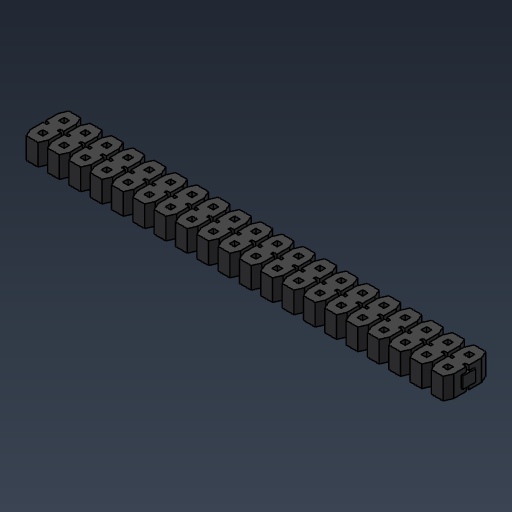
# Autodesk Inventor part: TSM-120-01-T-DV-P_body
Saved by Autodesk Inventor 2023.1 (Build 271208000, 208)
## iProperties
Category: PARTsolutions
Company: SAMTEC
Created: 2015-08-01
Part Number: TSM-120-01-T-DV-P_body
Catalog Web Link: www.cadenas.de
Description: TSM Series Body-TSM Series - (2,54 mm) .100" Surface Mount Terminal .025" Square Post Header
Vendor: SAMTEC
Document SubType Name: Modeling
Designer: PARTuser1
Manufacturer: SAMTEC
Mass: 0.492067 g
Surface Area: 13.1563 cm^2
Volume: 0.492067 cm^3
Density: 1 g/cm^3
Material: Allgemein
Appearance: PSOLRGB-127-127-127
PSOL_IDENT_0: {$CADENAS_DATA\23d-libs\samtec\modelling\tsm\parts\tsm_body.prj},251 {VTYP=3D},{NB=TSM-120-01-T-DV-P
PSOL_IDENT_1: _body},{LINA=TSM-120-01-T-DV-P_body},{NN=TSM Series Body},{DATE=20.05.2015 13:50:20},{GEOMDATE=20.05
PSOL_IDENT_2: .2015 06:27:00},{VERSION=},{LINEID=10},{LINESUBID=-1},{WBVAR=POS,LS,ROW,PLOPT,LCOPT,AOPT,SLOPT,POLOP
PSOL_IDENT_3: T,POPT,TROPT,KOPT}  {NB=TSM-120-01-T-DV-P_body},{LINA=TSM-120-01-T-DV-P_body},{KT=DUMMY},{PN=TSM-120
PSOL_IDENT_4: -01-T-DV-P},{SERIES=TSM},{POS=20},{POSPN=20},{LS=-01},{LSALG= '-01','-01','-02','-02','-03','-03','-
PSOL_IDENT_5: 04','-04' ,'-05','-05 (Non-standard option -  Please contact SAMTEC)' },{ROW=-DV},{ROWALG= '-SV','-S
PSOL_IDENT_6: V - Single Vertical', '-SH','-SH - Single Horizontal', '-DV' ,'-DV - Double Vertical' ,'-DV-S' ,'-DV
PSOL_IDENT_7: -S - Double Vertical Molded End Shrouds (Non-standard option -  Please contact SAMTEC)', '-DH', '-DH
PSOL_IDENT_8: - Double Horizontal' ,  '-MT','-MT - Mixed Technology','-EM','-EM - Edge Mount', '-TM','-TM - Tripl
PSOL_IDENT_9: e Mixed Technology'  },{PLOPT=-T},{PLOPTALG= '-T','-T - Matte Tin on Entire Pin','-S','-S - 30micro\
PSOL_IDENT_10: " Selective Gold in Contact Area, Matte Tin on Tail','-G','-G - 10micro\" Selective Gold in Contact
PSOL_IDENT_11: Area, 3micro\" Selective Gold on Tail','-L','-L - 10micro\" Selective Gold in Contact Area, Matte Ti
PSOL_IDENT_12: n on Tail','-TL','-TL - Tin/Lead (90/10) on Entire Pin','-STL','-STL - 30micro\" Selective Gold in C
PSOL_IDENT_13: ontact Area, Tin/Lead (90/10) on Tail','-F','-F - 3micro\" Selective Gold in Contact Area, Matte Tin
PSOL_IDENT_14: on Tail','-H','-H - 30micro\" Selective Gold in Contact Area, Matte Tin on Tail','-TM','-TM - Matte
PSOL_IDENT_15: Tin on Entire Pin','-SM','-SM - 30micro\" Selective Gold in Contact Area, Matte Tin on Tail','-LM','
PSOL_IDENT_16: -LM - 10micro\" Selective Gold in Contact Area, Matte Tin on Tail','-FM','-FM - 3micro\" Selective G
PSOL_IDENT_17: old in Contact Area, Matte Tin on Tail','-SS','-SS - 30micro\" Stripe Selective Gold in Contact Area
PSOL_IDENT_18: , Matte Tin on Tail' },{LCOPT=},{LCOPTALG= '','Not Selected','-LC','-LC - Locking Clip' },{AOPT=},{A
PSOL_IDENT_19: OPTALG= '','Not Selected','-A' , '-A - Alignment Pin'  },{SLOPT=},{SLOPTALG= '','Not Available' },{P
PSOL_IDENT_20: OLOPT=},{POLOPTALG= '','Not Selected','001','001','002','002','003','003','004','004','005','005','0
PSOL_IDENT_21: 06','006','007','007','008','008','009','009','010','010','011','011','012','012','013','013','014','
PSOL_IDENT_22: 014','015','015','016','016','017','017','018','018','019','019','020','020','021','021','022','022'
PSOL_IDENT_23: ,'023','023','024','024','025','025','026','026','027','027','028','028','029','029','030','030','03
PSOL_IDENT_24: 1','031','032','032','033','033','034','034','035','035','036','036','037','037','038','038','039','
PSOL_IDENT_25: 039','040','040' },{POLOPTMAX=480},{POLOPTMAX2='001','001','002','002','003','003','004','004','005'
PSOL_IDENT_26: ,'005','006','006','007','007','008','008','009','009','010','010','011','011','012','012','013','01
PSOL_IDENT_27: 3','014','014','015','015','016','016','017','017','018','018','019','019','020','020','021','021','
PSOL_IDENT_28: 022','022','023','023','024','024','025','025','026','026','027','027','028','028','029','029','030'
PSOL_IDENT_29: ,'030','031','031','032','032','033','033','034','034','035','035','036','036','037','037','038','03
PSOL_IDENT_30: 8','039','039','040','040'},{POLARIZE='001','001','002','002','003','003','004','004','005','005','0
PSOL_IDENT_31: 06','006','007','007','008','008','009','009','010','010','011','011','012','012','013','013','014','
PSOL_IDENT_32: 014','015','015','016','016','017','017','018','018','019','019','020','020','021','021','022','022'
PSOL_IDENT_33: ,'023','023','024','024','025','025','026','026','027','027','028','028','029','029','030','030','03
PSOL_IDENT_34: 1','031','032','032','033','033','034','034','035','035','036','036','037','037','038','038','039','
PSOL_IDENT_35: 039','040','040','041','041','042','042','043','043','044','044','045','045','046','046','047','047'
PSOL_IDENT_36: ,'048','048','049','049','050','050','051','051','052','052','053','053','054','054','055','055','05
PSOL_IDENT_37: 6','056','057','057','058','058','059','059','060','060','061','061','062','062','063','063','064','
PSOL_IDENT_38: 064','065','065','066','066','067','067','068','068','069','069','070','070','071','071','072','072'
PSOL_IDENT_39: ,'073','073','074','074','075','075','076','076','077','077','078','078','079','079','080','080','08
PSOL_IDENT_40: 1','081','082','082','083','083','084','084','085','085','086','086','087','087','088','088','089','
PSOL_IDENT_41: 089','090','090','091','091','092','092','093','093','094','094','095','095','096','096','097','097'
PSOL_IDENT_42: ,'098','098','099','099','100','100','101','101','102','102','103','103','104','104','105','105','10
PSOL_IDENT_43: 6','106','107','107','108','108','109','109','110','110','111','111','112','112','113','113','114','
PSOL_IDENT_44: 114','115','115','116','116','117','117','118','118','119','119','120','120','121','121','122','122'
PSOL_IDENT_45: ,'123','123','124','124','125','125','126','126','127','127','128','128','129','129','130','130','13
PSOL_IDENT_46: 1','131','132','132','133','133','134','134','135','135','136','136','137','137','138','138','139','
PSOL_IDENT_47: 139','140','140','141','141','142','142','143','143','144','144','145','145','146','146','147','147'
PSOL_IDENT_48: ,'148','148','149','149','150','150'},{POLOPTPN=},{POPT=-P},{POPTALG= '','Not Selected','-P','-P - P
PSOL_IDENT_49: ick & Place Pad' },{TROPT=},{TROPTALG= '','Not Selected','-TR','-TR - Tape & Reel' },{KOPT=},{KOPTAL
PSOL_IDENT_50: G= '','Not Available' },{BSH=0.230},{CSH=0.180},{ESH=0.1000},{ASH=0.9000},{RSH=2.00000},{SSH=0.90155
PSOL_IDENT_51: },{ASV=0.80000},{BSV=0.230},{CSV=0.280},{DMAXSV=0.208},{ESV=0.445},{FSV=0.165},{CDHMT=0.230},{BDVTM=
PSOL_IDENT_52: 0.23000},{CDV=0.30300},{DDV=0.28000},{GDV=0.80500}
NN: TSM Series Body
NT: TSM Series - (2,54 mm) .100" Surface Mount Terminal .025" Square Post Header
NB: TSM-120-01-T-DV-P_body
NBSYN: $PN._body
LINA: TSM-120-01-T-DV-P_body
SERIES: TSM
POS: 20
LS: -01
ROW: -DV - Double Vertical
PLOPT: -T - Matte Tin on Entire Pin
LCOPT: Not Selected
AOPT: Not Selected
SLOPT: Not Available
POLOPT: Not Selected
POPT: -P - Pick & Place Pad
TROPT: Not Selected
KOPT: Not Available
SUPPLIER: SAMTEC
ARTICLENO: TSM-120-01-T-DV-P_body
BOMINFO: TSM-120-01-T-DV-P_body
CREATOR: CADENAS GmbH
Title: TSM-120-01-T-DV-P_body
Author: Cadenas PARTsolutions
Comments: TSM Series - (2,54 mm) .100" Surface Mount Terminal .025" Square Post Header
Autodesk Inventor part; units mm, degrees
sketch "Sketch_1" plane through (0, 0, 0) normal (1, 0, 0) x (0, 1, 0)
  line L0 (-0.6985, 0.762) -> (-0.6985, -0.762)
  line L1 (-0.6985, -0.762) -> (0.6985, -0.762)
  line L2 (0.6985, -0.762) -> (0.6985, 0.762)
  line L3 (0.6985, 0.762) -> (-0.6985, 0.762)
  constraints: 8 end point
extrude "Extrusion1" add sketch "Sketch_1" along normal mid plane 50.8
sketch "Sketch_2" plane through (0, 0, 0) normal (0, 1, 0) x (-1, 0, 0)
  line L0 (25.2095, 0.1461) -> (25.2095, 1.651)
  line L1 (25.2095, 1.651) -> (24.8285, 2.54)
  line L2 (24.8285, 2.54) -> (23.4315, 2.54)
  line L3 (23.4315, 2.54) -> (23.0505, 1.651)
  line L4 (23.0505, 1.651) -> (23.0505, 0.1461)
  line L5 (23.0505, 0.1461) -> (23.495, 0.1461)
  line L6 (23.495, 0.1461) -> (23.495, -0.1461)
  line L7 (23.495, -0.1461) -> (23.0505, -0.1461)
  line L8 (23.0505, -0.1461) -> (23.0505, -1.651)
  line L9 (23.0505, -1.651) -> (23.4315, -2.54)
  line L10 (23.4315, -2.54) -> (24.8285, -2.54)
  line L11 (24.8285, -2.54) -> (25.2095, -1.651)
  line L12 (25.2095, -1.651) -> (25.2095, -0.1461)
  line L13 (25.2095, -0.1461) -> (24.765, -0.1461)
  line L14 (24.765, -0.1461) -> (24.765, 0.1461)
  line L15 (24.765, 0.1461) -> (25.2095, 0.1461)
  line L16 (24.4475, 1.5875) -> (23.8125, 1.5875)
  line L17 (23.8125, 1.5875) -> (23.8125, 0.9525)
  line L18 (23.8125, 0.9525) -> (24.4475, 0.9525)
  line L19 (24.4475, 0.9525) -> (24.4475, 1.5875)
  line L20 (24.4475, -0.9525) -> (23.8125, -0.9525)
  line L21 (23.8125, -0.9525) -> (23.8125, -1.5875)
  line L22 (23.8125, -1.5875) -> (24.4475, -1.5875)
  line L23 (24.4475, -1.5875) -> (24.4475, -0.9525)
  constraints: 48 end point
extrude "Extrusion2" add sketch "Sketch_2" along normal mid plane 2.54
pattern_linear "Rectangular Pattern1" count 20 spacing 2.54 along (1, 0, 0) of "Extrusion2"
ref_plane "body_XY" through (0, 0, 0) normal (0, -1, 0) x (1, 0, 0)
ref_plane "body_YZ" through (0, 0, 0) normal (1, 0, 0) x (0, 0, 1)
ref_plane "body_ZX" through (0, 0, 0) normal (0, 0, 1) x (0, -1, 0)
ref_plane "pick_place_pad_XY" through (0, 8.382, 0) normal (0, 1, 0) x (1, 0, 0)
ref_plane "pick_place_pad_YZ" through (0, 8.382, 0) normal (1, 0, 0) x (0, 0, -1)
ref_plane "pick_place_pad_ZX" through (0, 8.382, 0) normal (0, 0, -1) x (0, 1, 0)
ref_plane "terminal_dv_XY" through (0, 0, 0) normal (0, 1, 0) x (1, 0, 0)
ref_plane "terminal_dv_YZ" through (0, 0, 0) normal (1, 0, 0) x (0, 0, -1)
ref_plane "terminal_dv_ZX" through (0, 0, 0) normal (0, 0, -1) x (0, 1, 0)
body "Solid1"
